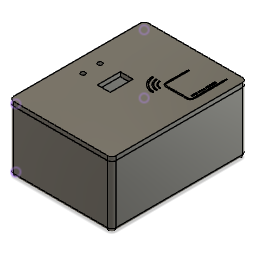
Boitier projet serrure rfid v10 (Autodesk Fusion 360 design; units mm, degrees)
Autodesk Fusion 360 part; units mm, degrees
note: some values were not read from the file. Chosen so that the rebuilt part matches the saved one: that a step has no effect.
(part 1 of 3)
sketch "Esquisse1" plane through (0, 0, 0) normal (0, 1, 0) x (1, 0, 0)
  line L0 (0, 0) -> (100, 0)
  line L1 (100, 0) -> (100, -130)
  line L2 (100, -130) -> (0, -130)
  line L3 (0, -130) -> (0, 0)
  dimension "d1" = 100
  dimension "d2" = 130
  constraint horizontal L0
  constraint vertical L1
  constraint horizontal L2
  constraint vertical L3
  constraint coincident L0.start L3.end
  measures "d1" distance of L0.start L0.end
  measures "d2" distance of L0.start L2.end
extrude "Extrusion1" add sketch "Esquisse1" along normal blind 65 makes body 1
extrude "Extrusion2" add 1 faces at (33.3333, 21.6667, 0) along direction (0, 0, -1) blind 10 on bodies 1 bodies 1
extrude "Extrusion3" add 1 faces at (100, 21.6667, 36.6667) along direction (1, 0, 0) blind 10 on bodies 1 bodies 1
extrude "Extrusion4" add 1 faces at (110, 21.6667, 36.6667) along direction (1, 0, 0) blind 10 on bodies 1 bodies 1
extrude "Extrusion5" add 1 faces at (80, 43.3333, 130) along direction (0, 0, 1) blind 10 on bodies 1 bodies 1
shell "Coque2" thickness 4 removed faces 1 at (40, 65, 90) on bodies 1
sketch "Esquisse3" plane through (0, 0, 0) normal (0, 1, 0) x (1, 0, 0)
  line L0 (-220, 0) -> (-100, 0)
  line L1 (-100, 0) -> (-100, -150)
  line L2 (-100, -150) -> (-220, -150)
  line L3 (-220, -150) -> (-220, 0)
  dimension "d15" = 150
  constraint horizontal L0
  constraint vertical L1
  constraint horizontal L2
  constraint vertical L3
  measures "d15" distance of L0.start L2.end
extrude "Extrusion6" add sketch "Esquisse3" along normal blind 5 separate body makes body 2
sketch "Esquisse5" plane through (0, 5, 0) normal (0, 1, 0) x (-1, 0, 0)
  line L0 (220, 150) -> (100, 150)
  line L1 (100, 150) -> (100, 0)
  line L2 (100, 0) -> (220, 0)
  line L3 (220, 0) -> (220, 150)
  line L4 (104.125, 145.875) -> (215.875, 145.875)
  line L5 (215.875, 145.875) -> (215.875, 4.125)
  line L6 (215.875, 4.125) -> (104.125, 4.125)
  line L7 (104.125, 4.125) -> (104.125, 145.875)
  line L8 (106.56, 6.625) -> (213.44, 6.625)
  line L9 (213.44, 6.625) -> (213.44, 143.375)
  line L10 (213.44, 143.375) -> (106.56, 143.375)
  line L11 (106.56, 143.375) -> (106.56, 6.625)
  point P0 (160, 75)
  point P1 (160, 75)
  dimension "d19" = 111.75
  dimension "d20" = 141.75
  dimension "d21" = 106.88
  dimension "d22" = 136.75
  constraint horizontal L4
  constraint perpendicular L4 L5
  constraint parallel L4 L6
  constraint parallel L5 L7
  constraint horizontal L8
  constraint perpendicular L8 L9
  constraint parallel L8 L10
  constraint parallel L9 L11
  constraint coincident P1 P0
  measures "d19" distance of L5.end L6.end
  measures "d20" distance of L4.end L5.end
  measures "d21" distance of L9.end L10.end
  measures "d22" distance of L8.end L9.end
extrude "Extrusion7" add sketch "Esquisse5" along normal blind 10 contours L4 L5 L6 L7 bodies 2
hole "Perçage1" at (4, 14.7265, 4.261) direction (-1, 0, 0) diameter 7.98 depth 5 tip angle 180 bodies 1
sketch "Esquisse9" plane through (0, 5, 0) normal (0, 1, 0) x (-1, 0, 0)
sketch "Esquisse10" plane through (0, 5, 0) normal (0, 1, 0) x (-1, 0, 0)
sketch "Esquisse11" plane through (0, 5, 0) normal (0, 1, 0) x (-1, 0, 0)
  circle A0 centre (117.4, 85) radius 2.6
  circle A1 centre (117.4, 65) radius 2.6
  dimension "d28" = 5.2
  dimension "d29" = 5.2
  measures "d28" diameter of A0
  measures "d29" diameter of A1
extrude "Extrusion8" cut sketch "Esquisse11" against normal blind 5 contours A0 bodies 2
sketch "Esquisse12" plane through (-138.697, 5, 40.8125) normal (0, 1, 0) x (-1, 0, 0)
  circle A0 centre (-21.303, 24.1872) radius 2.625
  dimension "d32" = 5.25
  measures "d32" diameter of A0
extrude "Extrusion9" cut sketch "Esquisse12" against normal blind 5 bodies 2
sketch "Esquisse15" plane through (0, 0, 0) normal (0, -1, 0) x (1, 0, 0)
  circle A0 centre (-117.3941, 64.9997) radius 2.625
  circle A1 centre (-117.4, 85) radius 2.6
  line L0 (-100, 150) -> (-220, 150)
  line L1 (-220, 150) -> (-220, 0)
  line L2 (-220, 0) -> (-100, 0)
  line L3 (-100, 0) -> (-100, 150)
  line L4 (-137.5, 61.625) -> (-152.5, 61.625)
  line L5 (-152.5, 61.625) -> (-152.5, 88.375)
  line L6 (-152.5, 88.375) -> (-137.5, 88.375)
  line L7 (-137.5, 88.375) -> (-137.5, 61.625)
  point P0 (-145, 75)
  dimension "d35" = 15
  dimension "d36" = 26.75
  constraint horizontal L4
  constraint perpendicular L4 L5
  constraint parallel L4 L6
  constraint parallel L5 L7
  measures "d35" distance of L5.end L6.end
  measures "d36" distance of L4.end L5.end
extrude "Extrusion10" cut sketch "Esquisse15" against normal blind 5 contours L4 L5 L6 L7 bodies 2
copy_body "Corps->Comp1" bodies 1 removing the originals makes body 3 in component "Component"
copy_body "Corps->Comp2" bodies 2 removing the originals makes body 4 in component "Component'"
mesh "Maillage1" [no effect]
mesh "Maillage2" [no effect]
mesh "Maillage3" [no effect]
sketch "Esquisse18" plane through (0, 0, 136) normal (0, 0, -1) x (-1, 0, 0)
  line L0 (-116, 4) -> (-4, 4)
  line L1 (-4, 4) -> (-4, 65)
  line L2 (-4, 65) -> (-116, 65)
  line L3 (-116, 65) -> (-116, 4)
  line L4 (-45.5271, 65) -> (-44.7886, 59.2457)
  constraint coincident L2 L4.start
extrude "Extrusion1'" add 1 faces at (118.6667, 65, 41.3333) along direction (0, 1, 0) blind 8 on bodies 3 bodies 3 in component "Component"
sketch "Esquisse19" plane through (0, 5, 0) normal (0, 1, 0) x (-1, 0, 0)
extrude "Extrusion2'" add 1 faces at (40, 48.6667, 140) along direction (0, 0, 1) blind 8 on bodies 3 bodies 3 in component "Component"
extrude "Extrusion3'" cut sketch "Esquisse18" against normal blind 8 bodies 3 in component "Component"
extrude "Extrusion4'" cut 1 faces at (78.6667, 70.3333, 136) along direction (0, 0, 1) blind 8 on bodies 3 bodies 3 in component "Component"
sketch "Esquisse20" plane through (0, 4, 0) normal (0, 1, 0) x (-1, 0, 0)
move_body "Déplacer1" bodies 4 to x (1, 0, 0) y (0, 1, 0) z (0, 0, 1) at (66.2703, -0.6856, 12.8538) in component "Component'"
move_body "Déplacer2" bodies 4 to x (-1, 0, 0) y (0, -1, 0) z (0, 0, 1) at (-213.12, 10, 0) in component "Component'"
extrude "Extrusion4''" add 1 faces at (-138.0153, -0.981, 158.7288) along direction (0, 0, 1) blind 4 on bodies 4 bodies 4 in component "Component'"
extrude "Extrusion5'" add 1 faces at (-139.3903, 9.019, 162.8538) along direction (0, 0, 1) blind 4 on bodies 4 bodies 4 in component "Component'"
extrude "Extrusion6'" add 1 faces at (-100.7653, 2.3523, 16.9788) along direction (0, 0, -1) blind 4 on bodies 4 bodies 4 in component "Component'"
extrude "Extrusion7'" add 1 faces at (-139.3903, 7.3523, 12.8538) along direction (0, 0, -1) blind 4 on bodies 4 bodies 4 in component "Component'"
move_body "Déplacer3" bodies 4 to x (1, 0, 0) y (0, 1, 0) z (0, 0, 1) at (178.6532, 79.1043, -18.6926) in component "Component'"
move_body "Déplacer4" bodies 4 to x (1, 0, 0) y (0, 1, 0) z (0, 0, 1) at (0.431, -11.6731, -0.2254) in component "Component'"
fillet "Congé1" radius 5 4 edges at (0, 36.5, -10) (120, 36.5, -10) (120, 36.5, 148) (0, 36.5, 148) on bodies 3 in component "Component"
fillet "Congé2" radius 5 8 edges at (120, 0, 69) (118.5355, 0, -8.5355) (60, 0, -10) (1.4645, 0, -8.5355) (0, 0, 69) (1.4645, 0, 146.5355) (60, 0, 148) (118.5355, 0, 146.5355) on bodies 3 in component "Component"
fillet "Congé1'" radius 5 4 edges at (119.6939, 75.6168, 147.9357) (-0.3061, 75.6168, 147.9357) (-0.3061, 75.6168, -10.0643) (119.6939, 75.6168, -10.0643) on bodies 4 in component "Component'"
move_body "Déplacer5" bodies 4 to x (1, 0, 0) y (0, 1, 0) z (0, 0, 1) at (0.4, 0, 0) in component "Component'"
sketch "Esquisse21" plane through (0, 78.1168, 0) normal (0, 1, 0) x (-1, 0, 0)
  arc A0 (-120.0939, -5.0643) -> (-115.0939, -10.0643) centre (-115.0939, -5.0643) ccw
  line L0 (-115.0939, -10.0643) -> (-5.0939, -10.0643)
  arc A1 (-5.0939, -10.0643) -> (-0.0939, -5.0643) centre (-5.0939, -5.0643) ccw
  line L1 (-0.0939, -5.0643) -> (-0.0939, 142.9357)
  arc A2 (-0.0939, 142.9357) -> (-5.0939, 147.9357) centre (-5.0939, 142.9357) ccw
  line L2 (-5.0939, 147.9357) -> (-115.0939, 147.9357)
  arc A3 (-115.0939, 147.9357) -> (-120.0939, 142.9357) centre (-115.0939, 142.9357) ccw
  line L3 (-120.0939, 142.9357) -> (-120.0939, -5.0643)
  line L4 (-52.5939, 55.5607) -> (-52.5939, 82.3107)
  line L5 (-52.5939, 82.3107) -> (-37.5939, 82.3107)
  line L6 (-37.5939, 82.3107) -> (-37.5939, 55.5607)
  line L7 (-37.5939, 55.5607) -> (-52.5939, 55.5607)
  circle A4 centre (-17.488, 58.9355) radius 2.625
  circle A5 centre (-17.4939, 78.9357) radius 2.6
  spline S0 degree 3 poles (-70.3957, 38.0285) (-70.0585, 36.7835) (-69.7723, 34.4433) (-69.8842, 34.1148) knots 0 0 0 0 1 1 1 1
  spline S1 degree 3 poles (-69.8842, 34.1148) (-69.9321, 34.0292) (-70.3145, 33.9241) (-70.7447, 33.9266) knots 0 0 0 0 1 1 1 1
  line L8 (-70.7447, 33.9266) -> (-71.5015, 33.8915)
  line L9 (-71.5015, 33.8915) -> (-71.5285, 34.6304)
  spline S2 degree 3 poles (-71.5285, 34.6304) (-71.557, 35.9049) (-72.1142, 38.0822) (-72.8294, 39.696) knots 0 0 0 0 1 1 1 1
  spline S3 degree 3 poles (-72.8294, 39.696) (-74.808, 44.161) (-79.4743, 47.4779) (-84.2893, 47.7898) knots 0 0 0 0 1 1 1 1
  spline S4 degree 3 poles (-84.2893, 47.7898) (-85.8385, 47.897) (-85.8903, 47.917) (-85.9175, 48.4627) knots 0 0 0 0 1 1 1 1
  spline S5 degree 3 poles (-85.9175, 48.4627) (-85.9701, 49.5979) (-85.8884, 49.6555) (-84.2953, 49.5463) knots 0 0 0 0 1 1 1 1
  spline S6 degree 3 poles (-84.2953, 49.5463) (-83.4988, 49.4916) (-82.4873, 49.3392) (-82.0892, 49.2153) knots 0 0 0 0 1 1 1 1
  spline S7 degree 3 poles (-82.0892, 49.2153) (-81.6731, 49.0993) (-80.9803, 48.8914) (-80.5542, 48.8014) knots 0 0 0 0 1 1 1 1
  spline S8 degree 3 poles (-80.5542, 48.8014) (-78.8182, 48.3693) (-75.5345, 46.2847) (-74.1144, 44.7258) knots 0 0 0 0 1 1 1 1
  spline S9 degree 3 poles (-74.1144, 44.7258) (-73.7723, 44.3411) (-73.2174, 43.6216) (-72.8714, 43.1313) knots 0 0 0 0 1 1 1 1
  spline S10 degree 3 poles (-72.8714, 43.1313) (-72.5255, 42.6411) (-72.1298, 42.087) (-72.0065, 41.9056) knots 0 0 0 0 1 1 1 1
  spline S11 degree 3 poles (-72.0065, 41.9056) (-71.5373, 41.234) (-70.6911, 39.2277) (-70.3957, 38.0285) knots 0 0 0 0 1 1 1 1
  spline S12 degree 3 poles (-74.3496, 35.3325) (-74.1797, 34.0777) (-74.2117, 33.9562) (-74.618, 33.9049) knots 0 0 0 0 1 1 1 1
  spline S13 degree 3 poles (-74.618, 33.9049) (-75.3869, 33.8002) (-75.5122, 33.9377) (-75.6821, 35.1925) knots 0 0 0 0 1 1 1 1
  spline S14 degree 3 poles (-75.6821, 35.1925) (-75.9371, 36.8815) (-77.0298, 39.2506) (-78.1159, 40.4426) knots 0 0 0 0 1 1 1 1
  spline S15 degree 3 poles (-78.1159, 40.4426) (-79.904, 42.3962) (-82.0655, 43.4978) (-84.5745, 43.7375) knots 0 0 0 0 1 1 1 1
  spline S16 degree 3 poles (-84.5745, 43.7375) (-85.2734, 43.814) (-85.8488, 43.9022) (-85.8568, 43.9202) knots 0 0 0 0 1 1 1 1
  spline S17 degree 3 poles (-85.8568, 43.9202) (-85.9601, 44.1533) (-85.8455, 45.1051) (-85.72, 45.1607) knots 0 0 0 0 1 1 1 1
  spline S18 degree 3 poles (-85.72, 45.1607) (-85.2538, 45.3673) (-83.2049, 45.0524) (-81.8055, 44.557) knots 0 0 0 0 1 1 1 1
  spline S19 degree 3 poles (-81.8055, 44.557) (-77.7186, 43.1286) (-74.9622, 39.7163) (-74.3496, 35.3325) knots 0 0 0 0 1 1 1 1
  spline S20 degree 3 poles (-78.2216, 34.7751) (-78.1607, 34.0083) (-78.2944, 33.7775) (-78.7922, 33.8358) knots 0 0 0 0 1 1 1 1
  spline S21 degree 3 poles (-78.7922, 33.8358) (-79.0451, 33.8739) (-79.1086, 34.0173) (-79.1836, 34.6706) knots 0 0 0 0 1 1 1 1
  spline S22 degree 3 poles (-79.1836, 34.6706) (-79.2781, 35.6585) (-80.0091, 37.3082) (-80.7013, 38.0955) knots 0 0 0 0 1 1 1 1
  spline S23 degree 3 poles (-80.7013, 38.0955) (-81.5526, 39.0484) (-82.9537, 39.8863) (-84.1881, 40.1545) knots 0 0 0 0 1 1 1 1
  spline S24 degree 3 poles (-84.1881, 40.1545) (-84.8053, 40.2886) (-85.4166, 40.361) (-85.5242, 40.3133) knots 0 0 0 0 1 1 1 1
  spline S25 degree 3 poles (-85.5242, 40.3133) (-85.7573, 40.21) (-85.9341, 40.5607) (-85.8699, 40.9967) knots 0 0 0 0 1 1 1 1
  spline S26 degree 3 poles (-85.8699, 40.9967) (-85.8298, 41.2934) (-85.6963, 41.3311) (-84.9874, 41.2805) knots 0 0 0 0 1 1 1 1
  spline S27 degree 3 poles (-84.9874, 41.2805) (-84.1033, 41.2218) (-82.2698, 40.6184) (-81.4857, 40.1078) knots 0 0 0 0 1 1 1 1
  spline S28 degree 3 poles (-81.4857, 40.1078) (-79.9852, 39.1423) (-78.3532, 36.4759) (-78.2216, 34.7751) knots 0 0 0 0 1 1 1 1
  spline S29 degree 3 poles (-83.5175, 26.8291) (-83.5431, 23.4496) (-83.5628, 20.0084) (-83.5657, 19.1919) knots 0 0 0 0 1 1 1 1
  spline S30 degree 3 poles (-83.5657, 19.1919) (-83.5786, 18.3496) (-83.6099, 15.225) (-83.6171, 12.2399) knots 0 0 0 0 1 1 1 1
  spline S31 degree 3 poles (-83.6171, 12.2399) (-83.6501, 7.57) (-83.7127, 6.7914) (-84.0534, 6.6404) knots 0 0 0 0 1 1 1 1
  spline S32 degree 3 poles (-84.0534, 6.6404) (-84.5734, 6.41) (-85.0869, 6.6973) (-85.148, 7.2709) knots 0 0 0 0 1 1 1 1
  spline S33 degree 3 poles (-85.148, 7.2709) (-85.1895, 7.5099) (-85.1824, 8.6072) (-85.1672, 9.6865) knots 0 0 0 0 1 1 1 1
  spline S34 degree 3 poles (-85.1672, 9.6865) (-85.1073, 11.7297) (-85.061, 17.6283) (-85.021, 25.0902) knots 0 0 0 0 1 1 1 1
  spline S35 degree 3 poles (-85.021, 25.0902) (-85.0223, 27.5138) (-84.9994, 30.2699) (-84.9825, 31.1999) knots 0 0 0 0 1 1 1 1
  spline S36 degree 3 poles (-84.9825, 31.1999) (-84.9275, 34.0774) (-85.7271, 35.0103) (-88.1368, 34.9293) knots 0 0 0 0 1 1 1 1
  spline S37 degree 3 poles (-88.1368, 34.9293) (-88.8757, 34.9022) (-90.0009, 34.8756) (-90.6501, 34.8882) knots 0 0 0 0 1 1 1 1
  spline S38 degree 3 poles (-90.6501, 34.8882) (-94.1092, 34.9) (-99.5558, 34.8462) (-110.5905, 34.7188) knots 0 0 0 0 1 1 1 1
  spline S39 degree 3 poles (-110.5905, 34.7188) (-112.5243, 34.6771) (-113.3809, 34.3833) (-113.8957, 33.5116) knots 0 0 0 0 1 1 1 1
  spline S40 degree 3 poles (-113.8957, 33.5116) (-114.2688, 32.8528) (-114.2729, 32.7652) (-114.2633, 26.9343) knots 0 0 0 0 1 1 1 1
  spline S41 degree 3 poles (-114.2633, 26.9343) (-114.2715, 24.8712) (-114.25, 22.6925) (-114.2686, 22.105) knots 0 0 0 0 1 1 1 1
  spline S42 degree 3 poles (-114.2686, 22.105) (-114.2725, 20.3227) (-114.2693, 12.2793) (-114.2692, 3.2262) knots 0 0 0 0 1 1 1 1
  spline S43 degree 3 poles (-114.2692, 3.2262) (-114.2604, -1.4896) (-114.3066, -5.5003) (-114.3407, -5.6655) knots 0 0 0 0 1 1 1 1
  spline S44 degree 3 poles (-114.3407, -5.6655) (-114.4745, -6.0896) (-115.0284, -6.2921) (-115.4025, -6.0288) knots 0 0 0 0 1 1 1 1
  spline S45 degree 3 poles (-115.4025, -6.0288) (-115.7666, -5.7396) (-115.7432, -6.1798) (-115.7504, 1.776) knots 0 0 0 0 1 1 1 1
  spline S46 degree 3 poles (-115.7504, 1.776) (-115.7485, 5.4025) (-115.751, 10.4428) (-115.7562, 12.9719) knots 0 0 0 0 1 1 1 1
  spline S47 degree 3 poles (-115.7562, 12.9719) (-115.7434, 15.509) (-115.7376, 19.0299) (-115.7516, 20.8043) knots 0 0 0 0 1 1 1 1
  spline S48 degree 3 poles (-115.7516, 20.8043) (-115.7397, 22.5687) (-115.738, 26.0019) (-115.7493, 28.3996) knots 0 0 0 0 1 1 1 1
  spline S49 degree 3 poles (-115.7493, 28.3996) (-115.7778, 33.2568) (-115.5836, 34.2224) (-114.3319, 35.2705) knots 0 0 0 0 1 1 1 1
  spline S50 degree 3 poles (-114.3319, 35.2705) (-113.3831, 36.0342) (-112.6819, 36.1947) (-109.7047, 36.2054) knots 0 0 0 0 1 1 1 1
  spline S51 degree 3 poles (-109.7047, 36.2054) (-108.3346, 36.2119) (-106.6916, 36.232) (-106.0583, 36.2552) knots 0 0 0 0 1 1 1 1
  spline S52 degree 3 poles (-106.0583, 36.2552) (-105.4171, 36.2605) (-103.9673, 36.2808) (-102.8521, 36.2816) knots 0 0 0 0 1 1 1 1
  spline S53 degree 3 poles (-102.8521, 36.2816) (-101.7369, 36.2824) (-100.2433, 36.3007) (-99.5403, 36.3118) knots 0 0 0 0 1 1 1 1
  spline S54 degree 3 poles (-99.5403, 36.3118) (-98.8373, 36.323) (-97.6862, 36.3397) (-96.9673, 36.315) knots 0 0 0 0 1 1 1 1
  spline S55 degree 3 poles (-96.9673, 36.315) (-96.2564, 36.3083) (-93.779, 36.3334) (-91.459, 36.3747) knots 0 0 0 0 1 1 1 1
  spline S56 degree 3 poles (-91.459, 36.3747) (-85.7554, 36.478) (-84.6744, 36.1204) (-83.8702, 33.9668) knots 0 0 0 0 1 1 1 1
  spline S57 degree 3 poles (-83.8702, 33.9668) (-83.5664, 33.136) (-83.5041, 31.8335) (-83.5175, 26.8291) knots 0 0 0 0 1 1 1 1
  spline S58 degree 3 poles (-110.6158, 29.8378) (-110.6663, 29.1289) (-111.059, 28.8047) (-111.4111, 29.1636) knots 0 0 0 0 1 1 1 1
  spline S59 degree 3 poles (-111.4111, 29.1636) (-111.5543, 29.2932) (-111.871, 29.2816) (-112.2196, 29.1485) knots 0 0 0 0 1 1 1 1
  line L10 (-112.2196, 29.1485) -> (-112.7835, 28.9201)
  line L11 (-112.7835, 28.9201) -> (-112.325, 29.3378)
  spline S60 degree 3 poles (-112.325, 29.3378) (-111.709, 29.9326) (-111.7026, 30.2572) (-112.2881, 30.3196) knots 0 0 0 0 1 1 1 1
  spline S61 degree 3 poles (-112.2881, 30.3196) (-113.0228, 30.3801) (-112.3873, 30.6403) (-111.4294, 30.6572) knots 0 0 0 0 1 1 1 1
  spline S62 degree 3 poles (-111.4294, 30.6572) (-110.5512, 30.6602) (-110.5671, 30.6961) (-110.6158, 29.8378) knots 0 0 0 0 1 1 1 1
  spline S63 degree 3 poles (-110.7381, 27.2092) (-110.774, 27.1933) (-110.8335, 27.4244) (-110.8551, 27.7152) knots 0 0 0 0 1 1 1 1
  spline S64 degree 3 poles (-110.8551, 27.7152) (-110.8842, 28.4102) (-110.8921, 28.4282) (-111.2149, 28.2851) knots 0 0 0 0 1 1 1 1
  spline S65 degree 3 poles (-111.2149, 28.2851) (-111.3404, 28.2295) (-111.492, 27.9907) (-111.5202, 27.7637) knots 0 0 0 0 1 1 1 1
  spline S66 degree 3 poles (-111.5202, 27.7637) (-111.5803, 27.4153) (-111.6062, 27.4253) (-111.6934, 27.8157) knots 0 0 0 0 1 1 1 1
  spline S67 degree 3 poles (-111.6934, 27.8157) (-111.7408, 28.1164) (-111.9179, 28.274) (-112.2246, 28.2882) knots 0 0 0 0 1 1 1 1
  spline S68 degree 3 poles (-112.2246, 28.2882) (-112.8897, 28.3367) (-112.6783, 28.5377) (-111.8757, 28.6144) knots 0 0 0 0 1 1 1 1
  spline S69 degree 3 poles (-111.8757, 28.6144) (-110.7385, 28.7108) (-110.5673, 28.615) (-110.6279, 27.8802) knots 0 0 0 0 1 1 1 1
  spline S70 degree 3 poles (-110.6279, 27.8802) (-110.6442, 27.5298) (-110.7023, 27.2251) (-110.7381, 27.2092) knots 0 0 0 0 1 1 1 1
  spline S71 degree 3 poles (-110.6611, 26.5998) (-110.9122, 26.4885) (-112.7522, 26.5742) (-112.6943, 26.6856) knots 0 0 0 0 1 1 1 1
  spline S72 degree 3 poles (-112.6943, 26.6856) (-112.6144, 26.8927) (-110.7483, 26.9902) (-110.6609, 26.7929) knots 0 0 0 0 1 1 1 1
  spline S73 degree 3 poles (-110.6609, 26.7929) (-110.6212, 26.7033) (-110.6253, 26.6157) (-110.6611, 26.5998) knots 0 0 0 0 1 1 1 1
  spline S74 degree 3 poles (-110.7924, 24.9112) (-110.9919, 24.5868) (-111.2171, 24.4656) (-111.6134, 24.4401) knots 0 0 0 0 1 1 1 1
  spline S75 degree 3 poles (-111.6134, 24.4401) (-112.2646, 24.4089) (-112.6744, 24.8495) (-112.6676, 25.5604) knots 0 0 0 0 1 1 1 1
  spline S76 degree 3 poles (-112.6676, 25.5604) (-112.6631, 26.0344) (-112.5894, 26.11) (-112.1672, 26.1255) knots 0 0 0 0 1 1 1 1
  spline S77 degree 3 poles (-112.1672, 26.1255) (-111.8943, 26.1391) (-111.4363, 26.1705) (-111.1634, 26.1841) knots 0 0 0 0 1 1 1 1
  spline S78 degree 3 poles (-111.1634, 26.1841) (-110.5301, 26.2073) (-110.3576, 25.5758) (-110.7924, 24.9112) knots 0 0 0 0 1 1 1 1
  spline S79 degree 3 poles (-110.5863, 22.1707) (-110.6562, 21.9896) (-110.8317, 21.8046) (-110.9751, 21.741) knots 0 0 0 0 1 1 1 1
  spline S80 degree 3 poles (-110.9751, 21.741) (-111.2341, 21.6477) (-111.2321, 21.6915) (-111.0505, 22.0079) knots 0 0 0 0 1 1 1 1
  spline S81 degree 3 poles (-111.0505, 22.0079) (-110.7432, 22.5732) (-111.0851, 23.1511) (-111.6687, 23.0641) knots 0 0 0 0 1 1 1 1
  spline S82 degree 3 poles (-111.6687, 23.0641) (-112.3419, 22.9374) (-112.5235, 22.6209) (-112.1775, 22.1306) knots 0 0 0 0 1 1 1 1
  spline S83 degree 3 poles (-112.1775, 22.1306) (-112.0045, 21.8855) (-112.0027, 21.7361) (-112.1441, 21.7164) knots 0 0 0 0 1 1 1 1
  spline S84 degree 3 poles (-112.1441, 21.7164) (-112.8412, 21.6435) (-112.8456, 23.0574) (-112.1284, 23.3752) knots 0 0 0 0 1 1 1 1
  spline S85 degree 3 poles (-112.1284, 23.3752) (-111.3752, 23.709) (-110.3167, 22.8694) (-110.5863, 22.1707) knots 0 0 0 0 1 1 1 1
  spline S86 degree 3 poles (-111.2875, 20.1223) (-111.6641, 19.9554) (-112.1621, 19.8206) (-112.3991, 19.8228) knots 0 0 0 0 1 1 1 1
  spline S87 degree 3 poles (-112.3991, 19.8228) (-112.8034, 19.8153) (-112.8113, 19.8332) (-112.4347, 20.0001) knots 0 0 0 0 1 1 1 1
  spline S88 degree 3 poles (-112.4347, 20.0001) (-111.9765, 20.2246) (-112.0035, 20.9635) (-112.4673, 21.187) knots 0 0 0 0 1 1 1 1
  spline S89 degree 3 poles (-112.4673, 21.187) (-113.1022, 21.5063) (-112.5148, 21.4878) (-111.6687, 21.1762) knots 0 0 0 0 1 1 1 1
  spline S90 degree 3 poles (-111.6687, 21.1762) (-110.546, 20.7727) (-110.4368, 20.4778) (-111.2875, 20.1223) knots 0 0 0 0 1 1 1 1
  spline S91 degree 3 poles (-110.9155, 17.9273) (-111.0869, 17.8299) (-111.3418, 17.8242) (-111.503, 17.9459) knots 0 0 0 0 1 1 1 1
  spline S92 degree 3 poles (-111.503, 17.9459) (-111.6642, 18.0675) (-112.0067, 18.0659) (-112.2836, 17.9647) knots 0 0 0 0 1 1 1 1
  spline S93 degree 3 poles (-112.2836, 17.9647) (-112.5705, 17.8375) (-112.684, 17.8516) (-112.5465, 17.9769) knots 0 0 0 0 1 1 1 1
  spline S94 degree 3 poles (-112.5465, 17.9769) (-112.4269, 18.0943) (-112.1597, 18.3628) (-111.9484, 18.5637) knots 0 0 0 0 1 1 1 1
  line L12 (-111.9484, 18.5637) -> (-111.5796, 18.9417)
  line L13 (-111.5796, 18.9417) -> (-112.1868, 19.1017)
  line L14 (-112.1868, 19.1017) -> (-112.8019, 19.2796)
  line L15 (-112.8019, 19.2796) -> (-112.2622, 19.3686)
  spline S95 degree 3 poles (-112.2622, 19.3686) (-111.9694, 19.434) (-111.4754, 19.4813) (-111.1847, 19.5028) knots 0 0 0 0 1 1 1 1
  spline S96 degree 3 poles (-111.1847, 19.5028) (-110.6828, 19.5322) (-110.649, 19.5043) (-110.6357, 18.8451) knots 0 0 0 0 1 1 1 1
  spline S97 degree 3 poles (-110.6357, 18.8451) (-110.6182, 18.4667) (-110.7521, 18.0426) (-110.9155, 17.9273) knots 0 0 0 0 1 1 1 1
  spline S98 degree 3 poles (-110.6124, 16.5171) (-110.6548, 15.9834) (-111.5255, 15.5761) (-112.1127, 15.7878) knots 0 0 0 0 1 1 1 1
  spline S99 degree 3 poles (-112.1127, 15.7878) (-112.5347, 15.9655) (-112.8247, 16.7166) (-112.6529, 17.2004) knots 0 0 0 0 1 1 1 1
  spline S100 degree 3 poles (-112.6529, 17.2004) (-112.533, 17.5109) (-110.8383, 17.511) (-110.7032, 17.2062) knots 0 0 0 0 1 1 1 1
  spline S101 degree 3 poles (-110.7032, 17.2062) (-110.6397, 17.0627) (-110.6101, 16.754) (-110.6124, 16.5171) knots 0 0 0 0 1 1 1 1
  spline S102 degree 3 poles (-110.8132, 13.1458) (-110.8711, 13.0343) (-111.1339, 13.0465) (-111.3848, 13.1285) knots 0 0 0 0 1 1 1 1
  spline S103 degree 3 poles (-111.3848, 13.1285) (-111.6436, 13.2283) (-112.014, 13.1929) (-112.2492, 13.0458) knots 0 0 0 0 1 1 1 1
  spline S104 degree 3 poles (-112.2492, 13.0458) (-112.5022, 12.8907) (-112.6516, 12.8889) (-112.6355, 13.0462) knots 0 0 0 0 1 1 1 1
  spline S105 degree 3 poles (-112.6355, 13.0462) (-112.6114, 13.1856) (-112.4539, 13.3626) (-112.2746, 13.4421) knots 0 0 0 0 1 1 1 1
  spline S106 degree 3 poles (-112.2746, 13.4421) (-112.0953, 13.5216) (-111.8999, 13.7583) (-111.8459, 13.9753) knots 0 0 0 0 1 1 1 1
  spline S107 degree 3 poles (-111.8459, 13.9753) (-111.7519, 14.2958) (-111.7937, 14.3417) (-112.1562, 14.2883) knots 0 0 0 0 1 1 1 1
  spline S108 degree 3 poles (-112.1562, 14.2883) (-112.5904, 14.2032) (-112.8948, 14.4544) (-112.5541, 14.6054) knots 0 0 0 0 1 1 1 1
  spline S109 degree 3 poles (-112.5541, 14.6054) (-112.4465, 14.6531) (-111.9626, 14.6745) (-111.4807, 14.652) knots 0 0 0 0 1 1 1 1
  spline S110 degree 3 poles (-111.4807, 14.652) (-110.6224, 14.6033) (-110.6145, 14.5854) (-110.653, 13.9461) knots 0 0 0 0 1 1 1 1
  spline S111 degree 3 poles (-110.653, 13.9461) (-110.6693, 13.5957) (-110.7474, 13.2393) (-110.8132, 13.1458) knots 0 0 0 0 1 1 1 1
  spline S112 degree 3 poles (-110.6819, 11.2518) (-110.7318, 11.1224) (-110.8015, 11.1344) (-110.873, 11.2958) knots 0 0 0 0 1 1 1 1
  spline S113 degree 3 poles (-110.873, 11.2958) (-110.9366, 11.4392) (-110.9423, 11.6941) (-110.8823, 11.8494) knots 0 0 0 0 1 1 1 1
  spline S114 degree 3 poles (-110.8823, 11.8494) (-110.7725, 12.1341) (-111.0549, 12.4809) (-111.3239, 12.3617) knots 0 0 0 0 1 1 1 1
  spline S115 degree 3 poles (-111.3239, 12.3617) (-111.3956, 12.3299) (-111.4616, 12.0432) (-111.4759, 11.7365) knots 0 0 0 0 1 1 1 1
  spline S116 degree 3 poles (-111.4759, 11.7365) (-111.4643, 11.4199) (-111.5362, 11.1949) (-111.6139, 11.2249) knots 0 0 0 0 1 1 1 1
  spline S117 degree 3 poles (-111.6139, 11.2249) (-111.6915, 11.2549) (-111.7431, 11.468) (-111.7229, 11.7129) knots 0 0 0 0 1 1 1 1
  spline S118 degree 3 poles (-111.7229, 11.7129) (-111.6986, 12.0455) (-111.7801, 12.181) (-112.0489, 12.2549) knots 0 0 0 0 1 1 1 1
  spline S119 degree 3 poles (-112.0489, 12.2549) (-112.3435, 12.3389) (-112.4093, 12.2454) (-112.4039, 11.7973) knots 0 0 0 0 1 1 1 1
  spline S120 degree 3 poles (-112.4039, 11.7973) (-112.4181, 11.4906) (-112.4842, 11.2039) (-112.5738, 11.1642) knots 0 0 0 0 1 1 1 1
  spline S121 degree 3 poles (-112.5738, 11.1642) (-112.6635, 11.1245) (-112.713, 11.3814) (-112.6867, 11.7578) knots 0 0 0 0 1 1 1 1
  spline S122 degree 3 poles (-112.6867, 11.7578) (-112.6341, 12.5105) (-112.4248, 12.6676) (-111.3813, 12.6366) knots 0 0 0 0 1 1 1 1
  spline S123 degree 3 poles (-111.3813, 12.6366) (-110.6804, 12.6039) (-110.6386, 12.5581) (-110.6272, 12.0483) knots 0 0 0 0 1 1 1 1
  spline S124 degree 3 poles (-110.6272, 12.0483) (-110.6236, 11.7496) (-110.6399, 11.3991) (-110.6819, 11.2518) knots 0 0 0 0 1 1 1 1
  spline S125 degree 3 poles (-111.6716, 9.4187) (-112.622, 8.9976) (-113.1616, 9.1017) (-112.4023, 9.5669) knots 0 0 0 0 1 1 1 1
  spline S126 degree 3 poles (-112.4023, 9.5669) (-112.0854, 9.7717) (-112.0714, 9.8852) (-112.3636, 10.3993) knots 0 0 0 0 1 1 1 1
  line L16 (-112.3636, 10.3993) -> (-112.6955, 11.003)
  line L17 (-112.6955, 11.003) -> (-111.6683, 10.6215)
  spline S127 degree 3 poles (-111.6683, 10.6215) (-111.099, 10.4019) (-110.6452, 10.1524) (-110.6593, 10.0389) knots 0 0 0 0 1 1 1 1
  spline S128 degree 3 poles (-110.6593, 10.0389) (-110.6813, 9.9434) (-111.1337, 9.6571) (-111.6716, 9.4187) knots 0 0 0 0 1 1 1 1
  spline S129 degree 3 poles (-110.6593, 8.1511) (-110.7262, 7.0917) (-112.0927, 6.7865) (-112.5059, 7.7189) knots 0 0 0 0 1 1 1 1
  spline S130 degree 3 poles (-112.5059, 7.7189) (-112.9032, 8.6155) (-112.7436, 8.8364) (-111.6523, 8.891) knots 0 0 0 0 1 1 1 1
  spline S131 degree 3 poles (-111.6523, 8.891) (-111.1245, 8.9103) (-110.6685, 8.8979) (-110.6526, 8.862) knots 0 0 0 0 1 1 1 1
  spline S132 degree 3 poles (-110.6526, 8.862) (-110.6367, 8.8261) (-110.643, 8.5015) (-110.6593, 8.1511) knots 0 0 0 0 1 1 1 1
  spline S133 degree 3 poles (-110.7699, 5.399) (-110.8216, 5.419) (-110.8711, 5.6759) (-110.8927, 5.9667) knots 0 0 0 0 1 1 1 1
  spline S134 degree 3 poles (-110.8927, 5.9667) (-110.9296, 6.8729) (-111.4673, 6.8276) (-111.4843, 5.8977) knots 0 0 0 0 1 1 1 1
  spline S135 degree 3 poles (-111.4843, 5.8977) (-111.4906, 5.5731) (-111.5784, 5.384) (-111.6699, 5.4936) knots 0 0 0 0 1 1 1 1
  spline S136 degree 3 poles (-111.6699, 5.4936) (-111.7614, 5.6032) (-111.8368, 5.8702) (-111.8087, 6.0971) knots 0 0 0 0 1 1 1 1
  spline S137 degree 3 poles (-111.8087, 6.0971) (-111.7844, 6.4297) (-111.85, 6.5293) (-112.087, 6.5316) knots 0 0 0 0 1 1 1 1
  spline S138 degree 3 poles (-112.087, 6.5316) (-112.2722, 6.5139) (-112.4059, 6.283) (-112.4322, 5.9067) knots 0 0 0 0 1 1 1 1
  spline S139 degree 3 poles (-112.4322, 5.9067) (-112.5086, 5.2077) (-112.7393, 5.5346) (-112.6887, 6.2435) knots 0 0 0 0 1 1 1 1
  spline S140 degree 3 poles (-112.6887, 6.2435) (-112.6585, 6.5143) (-112.6384, 6.7592) (-112.6363, 6.803) knots 0 0 0 0 1 1 1 1
  spline S141 degree 3 poles (-112.6363, 6.803) (-112.6263, 6.8289) (-112.1762, 6.8782) (-111.6226, 6.8875) knots 0 0 0 0 1 1 1 1
  line L18 (-111.6226, 6.8875) -> (-110.6388, 6.8944)
  line L19 (-110.6388, 6.8944) -> (-110.6576, 6.1138)
  spline S142 degree 3 poles (-110.6576, 6.1138) (-110.668, 5.7016) (-110.7181, 5.379) (-110.7699, 5.399) knots 0 0 0 0 1 1 1 1
  spline S143 degree 3 poles (-110.6461, 3.9093) (-110.7799, 3.4852) (-111.3876, 3.2589) (-111.5386, 3.5996) knots 0 0 0 0 1 1 1 1
  spline S144 degree 3 poles (-111.5386, 3.5996) (-111.6339, 3.8148) (-111.7753, 3.795) (-112.148, 3.5226) knots 0 0 0 0 1 1 1 1
  spline S145 degree 3 poles (-112.148, 3.5226) (-112.4569, 3.2999) (-112.6621, 3.2304) (-112.7178, 3.3559) knots 0 0 0 0 1 1 1 1
  spline S146 degree 3 poles (-112.7178, 3.3559) (-112.7654, 3.4635) (-112.6079, 3.6406) (-112.3748, 3.7439) knots 0 0 0 0 1 1 1 1
  spline S147 degree 3 poles (-112.3748, 3.7439) (-112.1417, 3.8472) (-111.9025, 4.0819) (-111.8584, 4.273) knots 0 0 0 0 1 1 1 1
  spline S148 degree 3 poles (-111.8584, 4.273) (-111.7745, 4.5677) (-111.8501, 4.6415) (-112.2264, 4.6678) knots 0 0 0 0 1 1 1 1
  spline S149 degree 3 poles (-112.2264, 4.6678) (-113.0668, 4.7244) (-112.6423, 4.9769) (-111.6485, 5.0096) knots 0 0 0 0 1 1 1 1
  spline S150 degree 3 poles (-111.6485, 5.0096) (-110.6548, 5.0424) (-110.43, 4.7773) (-110.6461, 3.9093) knots 0 0 0 0 1 1 1 1
  spline S151 degree 3 poles (-111.1888, 30.3562) (-111.4596, 30.3864) (-111.6134, 29.9106) (-111.4386, 29.5161) knots 0 0 0 0 1 1 1 1
  spline S152 degree 3 poles (-111.4386, 29.5161) (-111.2956, 29.1933) (-110.8352, 29.4617) (-110.8607, 29.858) knots 0 0 0 0 1 1 1 1
  spline S153 degree 3 poles (-110.8607, 29.858) (-110.8841, 30.2981) (-110.8921, 30.316) (-111.1888, 30.3562) knots 0 0 0 0 1 1 1 1
  spline S154 degree 3 poles (-111.4167, 25.8359) (-112.2352, 25.795) (-112.4983, 25.614) (-112.3394, 25.2554) knots 0 0 0 0 1 1 1 1
  spline S155 degree 3 poles (-112.3394, 25.2554) (-112.0136, 24.5202) (-110.9719, 24.6385) (-110.9094, 25.4171) knots 0 0 0 0 1 1 1 1
  spline S156 degree 3 poles (-110.9094, 25.4171) (-110.8831, 25.7935) (-110.9587, 25.8672) (-111.4167, 25.8359) knots 0 0 0 0 1 1 1 1
  spline S157 degree 3 poles (-111.4063, 20.7776) (-111.5636, 20.7937) (-111.715, 20.7481) (-111.745, 20.6704) knots 0 0 0 0 1 1 1 1
  spline S158 degree 3 poles (-111.745, 20.6704) (-111.8348, 20.4375) (-111.5223, 20.3615) (-111.311, 20.5624) knots 0 0 0 0 1 1 1 1
  spline S159 degree 3 poles (-111.311, 20.5624) (-111.1455, 20.7216) (-111.1614, 20.7574) (-111.4063, 20.7776) knots 0 0 0 0 1 1 1 1
  spline S160 degree 3 poles (-111.181, 19.2041) (-111.4518, 19.2343) (-111.6057, 18.7585) (-111.4308, 18.364) knots 0 0 0 0 1 1 1 1
  spline S161 degree 3 poles (-111.4308, 18.364) (-111.3117, 18.095) (-111.0885, 18.1725) (-110.9288, 18.5865) knots 0 0 0 0 1 1 1 1
  spline S162 degree 3 poles (-110.9288, 18.5865) (-110.779, 18.9747) (-110.8584, 19.154) (-111.181, 19.2041) knots 0 0 0 0 1 1 1 1
  spline S163 degree 3 poles (-111.5159, 17.1035) (-112.2865, 17.1482) (-112.5636, 16.8537) (-112.2177, 16.3635) knots 0 0 0 0 1 1 1 1
  spline S164 degree 3 poles (-112.2177, 16.3635) (-111.9055, 15.9011) (-111.1526, 16.0417) (-110.9688, 16.5951) knots 0 0 0 0 1 1 1 1
  spline S165 degree 3 poles (-110.9688, 16.5951) (-110.8249, 17.045) (-110.8508, 17.055) (-111.5159, 17.1035) knots 0 0 0 0 1 1 1 1
  spline S166 degree 3 poles (-111.2321, 14.3331) (-111.519, 14.206) (-111.5119, 13.4154) (-111.2273, 13.3055) knots 0 0 0 0 1 1 1 1
  spline S167 degree 3 poles (-111.2273, 13.3055) (-111.0461, 13.2356) (-110.7983, 14.0319) (-110.9175, 14.3009) knots 0 0 0 0 1 1 1 1
  spline S168 degree 3 poles (-110.9175, 14.3009) (-110.9493, 14.3726) (-111.0887, 14.3967) (-111.2321, 14.3331) knots 0 0 0 0 1 1 1 1
  spline S169 degree 3 poles (-111.4576, 10.2429) (-111.6149, 10.259) (-111.7663, 10.2134) (-111.7963, 10.1358) knots 0 0 0 0 1 1 1 1
  spline S170 degree 3 poles (-111.7963, 10.1358) (-111.8862, 9.9029) (-111.5736, 9.8269) (-111.3623, 10.0278) knots 0 0 0 0 1 1 1 1
  spline S171 degree 3 poles (-111.3623, 10.0278) (-111.1968, 10.1869) (-111.2127, 10.2228) (-111.4576, 10.2429) knots 0 0 0 0 1 1 1 1
  spline S172 degree 3 poles (-111.6427, 8.5305) (-112.5768, 8.4598) (-112.6126, 8.4439) (-112.3901, 7.9419) knots 0 0 0 0 1 1 1 1
  spline S173 degree 3 poles (-112.3901, 7.9419) (-112.1994, 7.5115) (-111.8172, 7.4235) (-111.2075, 7.6936) knots 0 0 0 0 1 1 1 1
  spline S174 degree 3 poles (-111.2075, 7.6936) (-110.9564, 7.8049) (-110.8126, 8.2548) (-110.9397, 8.5417) knots 0 0 0 0 1 1 1 1
  spline S175 degree 3 poles (-110.9397, 8.5417) (-110.9477, 8.5596) (-111.2643, 8.548) (-111.6427, 8.5305) knots 0 0 0 0 1 1 1 1
  spline S176 degree 3 poles (-111.2606, 4.6667) (-111.6013, 4.5157) (-111.6078, 3.998) (-111.2755, 3.7805) knots 0 0 0 0 1 1 1 1
  spline S177 degree 3 poles (-111.2755, 3.7805) (-111.1143, 3.6589) (-111.0226, 3.7424) (-110.9466, 4.055) knots 0 0 0 0 1 1 1 1
  spline S178 degree 3 poles (-110.9466, 4.055) (-110.8325, 4.6204) (-110.9199, 4.8177) (-111.2606, 4.6667) knots 0 0 0 0 1 1 1 1
extrude "Extrusion9'" cut 1 faces at (77.9073, 69.7835, 137.3107) along direction (0, 0, 1) blind 1 on bodies 4 bodies 4 in component "Component'"
extrude "Extrusion10'" cut 1 faces at (42.2806, 69.7835, 0.5607) along direction (0, 0, -1) blind 1 on bodies 4 bodies 4 in component "Component'"
extrude "Extrusion11" add 1 faces at (113.5339, 66.4502, 92.0607) along direction (-1, 0, 0) blind 2.3 on bodies 4 bodies 4 in component "Component'"
extrude "Extrusion12" add 1 faces at (6.6539, 69.7835, 92.0607) along direction (1, 0, 0) blind 2.3 on bodies 4 bodies 4 in component "Component'"
sketch "Esquisse22" plane through (4, 0, 0) normal (1, 0, 0) x (0, 0, -1)
  line L0 (-144, 4) -> (6, 4)
  line L1 (6, 73) -> (-144, 73)